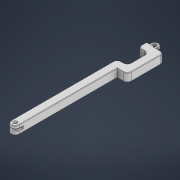
# Autodesk Inventor part: Support
Saved by Autodesk Inventor 2021 (Build 250183000, 183)
## iProperties
Created: 2021-01-30
Part Number: Support
Material: Generic
Document SubType Name: Modeling
Designer: PaisW
Density: 1 g/cm^3
Appearance: Default
Author: PaisW
Autodesk Inventor part; units mm, degrees
ref_plane "YZ Plane" through (0, 0, 0) normal (1, 0, 0) x (0, 1, 0)
ref_plane "XZ Plane" through (0, 0, 0) normal (0, 1, 0) x (-1, 0, 0)
ref_plane "XY Plane" through (0, 0, 0) normal (0, 0, 1) x (1, 0, 0)
sketch "Sketch4" plane through (0, 0, 0) normal (0, 1, 0) x (-1, 0, 0)
  circle A0 centre (0, 0) radius 8.5
  circle A1 centre (0, 0) radius 17
  line L0 (-17, -600) -> (17, -600)
  line L1 (17, -600) -> (17, 0)
  line L2 (17, 0) -> (-17, 0)
  line L3 (-17, 0) -> (-17, -600)
  line L4 (-17, -600) -> (17, 0) construction
  line L5 (17, -600) -> (-17, 0) construction
  circle A2 centre (0, -600) radius 17
  circle A3 centre (0, -600) radius 8.5
  line L6 (17, -422) -> (-61, -422)
  line L7 (-61, -422) -> (-61, -456)
  line L8 (-61, -456) -> (17, -456)
  line L9 (17, -456) -> (17, -422)
  line L10 (17, -580) -> (-61, -580)
  line L11 (-61, -580) -> (-61, -546)
  line L12 (-61, -546) -> (17, -546)
  line L13 (17, -546) -> (17, -580)
  line L14 (-61, -546) -> (-27, -546)
  line L15 (-27, -546) -> (-27, -456)
  line L16 (-27, -456) -> (-61, -456)
  line L17 (-61, -456) -> (-61, -546)
  point P0 (0, -300)
  point P1 (-17, 0)
  point P2 (17, -546)
  point P3 (17, -456)
  point P4 (-17, -422)
  point P5 (-17, -580)
  dimension "d14" = 34
  dimension "d13" = 17
  dimension "d15" = 600
  dimension "d24" = 20
  dimension "d25" = 34
  dimension "d26" = 90
  dimension "d27" = 10
  constraints: 36 end point, 8 parallel, 6 perpendicular, 4 horizontal, 4 point on line, 3 coincident, 3 midpoint, 2 centre point, 1 equal radius, 1 vertical, 6 other
  measures "d13" diameter of A0
  measures "d15" distance of point (0, -600) point (0, 0)
  measures "d24" distance from line of L10 point (0, -600)
  measures "d25" distance between parallel lines of L17 L15
  measures "d26" distance of L14.end L15.end
  measures "d27" distance between parallel lines of L3 L15
extrude "Extrusion4" add sketch "Sketch4" along normal blind 36 contours L2 A1 A0 | A0 L2 A1 | L1 L6 L3 A1 | L1 L8 L3 L6 | L3 L8 L7 L6 | L1 L10 L3 L12 | L3 L10 L11 L12 | L15 L12 L17 L8 | L1 A2 L3 L10 | A2 L0 A3 | L0 A3 A2
sketch "Sketch5" plane through (-17, 0, -600) normal (-1, 0, 0) x (0, 0, 1)
  line L0 (617, 0) -> (617, 36) projected
  line L1 (617, 24) -> (583, 24)
  line L2 (583, 24) -> (583, 12)
  line L3 (583, 12) -> (617, 12)
  line L4 (617, 12) -> (617, 24)
  line L5 (0, 36) -> (600, 36) projected
  line L6 (-17, 36) -> (17, 36)
  line L7 (17, 36) -> (17, 24)
  line L8 (17, 24) -> (-17, 24)
  line L9 (-17, 24) -> (-17, 36)
  line L10 (17, 24) -> (-17, 36) construction
  line L11 (-17, 24) -> (17, 36) construction
  line L12 (-17, 0) -> (-17, 36) projected
  line L13 (17, 12) -> (-17, 12)
  line L14 (-17, 12) -> (-17, 0)
  line L15 (-17, 0) -> (17, 0)
  line L16 (17, 0) -> (17, 12)
  line L17 (17, 12) -> (-17, 0) construction
  line L18 (-17, 12) -> (17, 0) construction
  line L19 (0, 0) -> (600, 0) projected
  point P0 (600, 24)
  point P1 (0, 30)
  point P2 (0, 6)
  dimension "d18" = 12
  dimension "d19" = 12
  constraints: 32 end point, 6 parallel, 4 midpoint, 3 collinear, 3 equal length, 3 horizontal, 3 perpendicular, 2 point on line, 2 vertical alignment
  measures "d18" distance of L1.end L2.end
  measures "d19" distance between parallel lines of L5 L1
extrude "Extrusion5" cut sketch "Sketch5" against normal through all
fillet "Fillet1" radius 2 4 edges at (0, 36, -583) (0, 0, -583) (0, 24, -583) (0, 12, -583)
fillet "Fillet2" radius 2 41 edges at (0, 0, 17) (17, 0, -580.5) (17, 0, -211) (17, 0.5858, -582.4142) (17, 6, -583) (17, 11.4142, -583.5858) (17, 12, -592.5) (0, 12, -617) (-17, 12, -592.5) (-17, 11.4142, -583.5858) (-17, 6, -583) (-17, 0.5858, -582.4142) (-17, 0, -563.5) (-17, 0, -228) (0, 36, 17) (17, 36, -580.5) (17, 36, -211) (17, 35.4142, -582.4142) (17, 30, -583) (17, 24.5858, -583.5858) (17, 24, -592.5) (12.0242, 24, -612.0174) (-12.0242, 24, -612.0174) (-17, 24, -592.5) (-17, 24.5858, -583.5858) (-17, 30, -583) (-17, 35.4142, -582.4142) (-17, 36, -563.5) (-17, 36, -228) (61, 0, -501) (39, 0, -422) (39, 0, -580) (39, 36, -580) (61, 36, -501) (39, 36, -422) (5, 36, -456) (5, 0, -456) (5, 36, -546) (5, 0, -546) (27, 36, -501) (27, 0, -501)
fillet "Fillet2" radius 16 6 edges at (-17, 18, -546) (27, 18, -546) (27, 18, -456) (-17, 18, -456) (61, 18, -422) (61, 18, -580)
body "Solid1"
body "Solid2"
